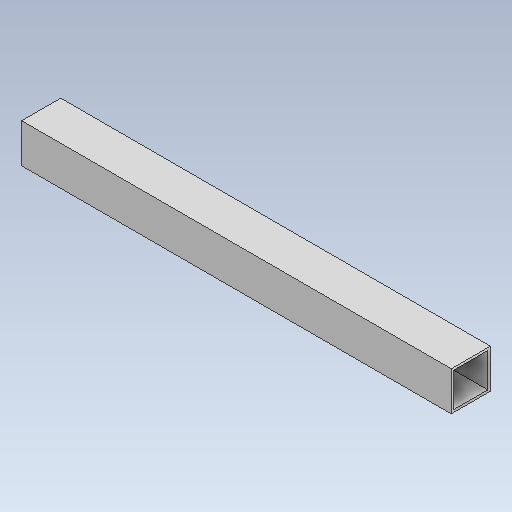
# Autodesk Inventor part: Part1-17-11in
Saved by Autodesk Inventor 2023 (Build 270158000, 158)
## iProperties
Created: 2023-03-16
Part Number: Part1-17-11in
Material: Generic
Document SubType Name: Modeling
Designer: mvp5338
Density: 1 g/cm^3
Appearance: Default
Author: mvp5338
Autodesk Inventor part; units mm, degrees
ref_plane "YZ Plane" through (0, 0, 0) normal (1, 0, 0) x (0, 1, 0)
ref_plane "XZ Plane" through (0, 0, 0) normal (0, 1, 0) x (-1, 0, 0)
ref_plane "XY Plane" through (0, 0, 0) normal (0, 0, 1) x (1, 0, 0)
sketch "Sketch1" plane through (0, 0, 0) normal (1, 0, 0) x (0, 1, 0)
  line L0 (12.7, 12.2788) -> (-12.7, 12.2788)
  line L1 (-12.7, 12.2788) -> (-12.7, -13.1212)
  line L2 (-12.7, -13.1212) -> (12.7, -13.1212)
  line L3 (12.7, -13.1212) -> (12.7, 12.2788)
  line L4 (0, 32.4321) -> (0, -31.5519)
  line L5 (24.3369, 0) -> (-19.9975, 0)
  point P0 (0, 0)
  dimension "d0" = 25.4
  constraints: 12 end point, 2 horizontal, 2 parallel, 2 perpendicular, 1 vertical, 1 other
  measures "d0" distance of L2.end L0.start
extrude "Extrusion1" add sketch "Sketch1" along normal blind 279.4
sketch "Sketch3" plane through (279.4, 0, 0) normal (1, 0, 0) x (0, 0, -1)
  line L0 (-10.6786, 11.1125) -> (11.521, 11.1125)
  line L1 (11.521, 11.1125) -> (11.521, -11.0998)
  line L2 (11.521, -11.0998) -> (-10.6786, -11.0998)
  line L3 (-10.6786, -11.0998) -> (-10.6786, 11.1125)
  line L4 (13.1212, 12.7) -> (-12.2788, 12.7) projected
  line L5 (-12.2788, 12.7) -> (-12.2788, -12.7) projected
  line L6 (13.1212, -12.7) -> (13.1212, 12.7) projected
  line L7 (-12.2788, -12.7) -> (13.1212, -12.7) projected
  point P0 (0, 0)
  dimension "d5" = 1.5875
  dimension "d6" = 1.6002
  dimension "d7" = 1.6002
  dimension "d8" = 1.6002
  constraints: 8 end point, 2 parallel, 1 horizontal, 1 perpendicular
  measures "d5" distance between parallel lines of L4 L0
  measures "d6" distance between parallel lines of L5 L3
  measures "d7" distance between parallel lines of L6 L1
  measures "d8" distance between parallel lines of L7 L2
extrude "Extrusion2" cut sketch "Sketch3" against normal through all contours L0 L1 L2 L3
body "Solid1"
